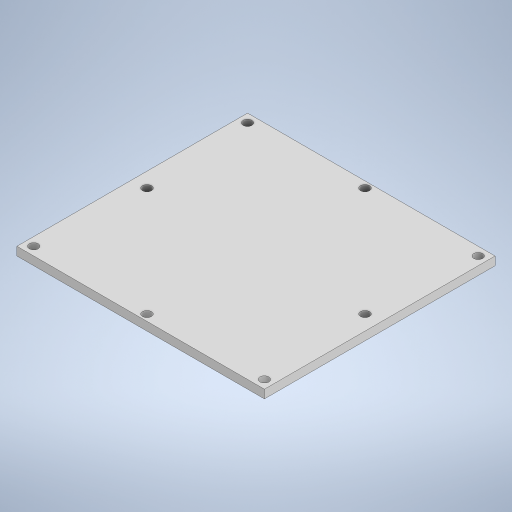
# Autodesk Inventor part: DummyBoard
Saved by Autodesk Inventor 2023 (Build 270158000, 158)
## iProperties
Created: 2022-08-17
Part Number: DummyBoard
Material: Generic
Document SubType Name: Modeling
Designer: Aditya Bansal
Density: 1 g/cm^3
Appearance: Default
Author: Aditya Bansal
Autodesk Inventor part; units mm, degrees
ref_plane "YZ Plane" through (0, 0, 0) normal (1, 0, 0) x (0, 1, 0)
ref_plane "XZ Plane" through (0, 0, 0) normal (0, 1, 0) x (-1, 0, 0)
ref_plane "XY Plane" through (0, 0, 0) normal (0, 0, 1) x (1, 0, 0)
sketch "Sketch1" plane through (0, 0, 0) normal (0, 1, 0) x (-1, 0, 0)
  line L0 (0, 0) -> (-88, 0)
  line L1 (-88, 0) -> (-88, -82)
  line L2 (-88, -82) -> (0, -82)
  line L3 (0, -82) -> (0, 0)
  line L4 (-2.25, -82.75) -> (-85.75, -82.75) construction
  line L5 (-85.75, -82.75) -> (-85.75, 0.75) construction
  line L6 (-85.75, 0.75) -> (-2.25, 0.75) construction
  line L7 (-2.25, 0.75) -> (-2.25, -82.75) construction
  circle A0 centre (-44, -79.75) radius 1.6
  circle A1 centre (-82.75, -41) radius 1.6
  circle A2 centre (-5.25, -41) radius 1.6
  circle A3 centre (-44, -2.25) radius 1.6
  circle A4 centre (-3, -79) radius 1.6
  circle A5 centre (-3, -3) radius 1.6
  circle A6 centre (-85, -3) radius 1.6
  circle A7 centre (-85, -79) radius 1.6
  dimension "d37" = 88
  dimension "d38" = 82
  dimension "d39" = 83.5
  dimension "d40" = 2.25
  dimension "d41" = 0.75
  dimension "d42" = 3.2
  dimension "d43" = 3
  dimension "d44" = 3
  dimension "d45" = 3
  dimension "d46" = 3
  dimension "d47" = 41
  dimension "d48" = 44
  dimension "d50" = 3.2
  dimension "d51" = 3
  dimension "d52" = 3
  dimension "d53" = 3
  dimension "d54" = 3
  constraints: 16 end point, 8 centre point, 6 equal radius, 4 parallel, 3 horizontal alignment, 3 perpendicular, 3 vertical alignment, 2 horizontal, 1 coincident
  measures "d37" distance of L1.end L2.end
  measures "d38" distance of L1.start L1.end
  measures "d39" distance of L4.start L5.start
  measures "d40" distance between parallel lines of L1 L5
  measures "d41" distance between parallel lines of L6 L0
  measures "d42" diameter of A1
  measures "d43" distance from line of A0.centre L4
  measures "d44" distance from line of L6 A3.centre
  measures "d45" distance from line of L7 A2.centre
  measures "d46" distance from line of L5 A1.centre
  measures "d47" distance from line of L2 A2.centre
  measures "d48" distance from line of L1 A3.centre
  measures "d50" diameter of A5
  measures "d51" distance from line of L3 A5.centre
  measures "d52" distance from line of L0 A5.centre
  measures "d53" distance from line of L1 A6.centre
  measures "d54" distance from line of L2 A4.centre
extrude "Extrusion1" add sketch "Sketch1" along normal blind 3
equation "\"d40\" = -0.5 * d39 + 0.5 * d37"
equation "\"d41\" = -0.5 * d38 + 0.5 * d39"
equation "\"d44\" = d43"
equation "\"d46\" = d45"
equation "\"d47\" = 0.5 * d38"
equation "\"d48\" = 0.5 * d37"
equation "\"d52\" = d51"
equation "\"d53\" = d51"
equation "\"d54\" = d52"
body "Solid1"
